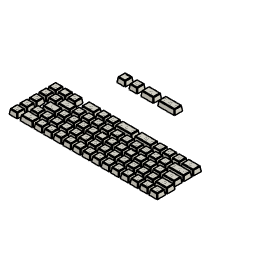
Launch Lite Keycaps v6 (Autodesk Fusion 360 design; units mm, degrees)
Autodesk Fusion 360 part; units mm, degrees
note: some values were not read from the file. Set by a fixed rule: which face or edge a step refers to.
sketch "Sketch1" plane through (0, 0, 0) normal (0, 0, 1) x (1, 0, 0)
  line L0 (-100, 50) -> (-82, 50)
  line L1 (-82, 50) -> (-82, 32)
  line L2 (-82, 32) -> (-100, 32)
  line L3 (-100, 32) -> (-100, 50)
  line L4 (-75, 50) -> (-57, 50)
  line L5 (-57, 50) -> (-57, 32)
  line L6 (-57, 32) -> (-75, 32)
  line L7 (-75, 32) -> (-75, 50)
  line L8 (-50, 50) -> (-23, 50)
  line L9 (-23, 50) -> (-23, 32)
  line L10 (-23, 32) -> (-50, 32)
  line L11 (-50, 32) -> (-50, 50)
  line L12 (-15, 50) -> (21, 50)
  line L13 (21, 50) -> (21, 32)
  line L14 (21, 32) -> (-15, 32)
  line L15 (-15, 32) -> (-15, 50)
  dimension "d1" = 18
  dimension "d2" = 18
  dimension "d3" = 18
  dimension "d4" = 18
  dimension "d5" = 27
  dimension "d6" = 18
  dimension "d7" = 36
  dimension "d8" = 18
  constraint horizontal L0
  constraint vertical L1
  constraint horizontal L2
  constraint vertical L3
  constraint horizontal L4
  constraint vertical L5
  constraint horizontal L6
  constraint vertical L7
  constraint horizontal L8
  constraint vertical L9
  constraint horizontal L10
  constraint vertical L11
  constraint horizontal L12
  constraint vertical L13
  constraint horizontal L14
  constraint vertical L15
  measures "d1" distance of L0.start L0.end
  measures "d2" distance of L0.start L2.end
  measures "d3" distance of L4.start L4.end
  measures "d4" distance of L4.start L6.end
  measures "d5" distance of L8.start L8.end
  measures "d6" distance of L8.start L10.end
  measures "d7" distance of L12.start L12.end
  measures "d8" distance of L12.start L14.end
extrude "Extrude1" add sketch "Sketch1" along normal blind 10 makes body 1 at (-41, 38, 0) makes body 2 at (-69, 44, 0) makes body 3 at (-3, 44, 0) makes body 4 at (-94, 44, 0)
shell "Shell1" thickness 1.75 removed faces 4 at (-41, 38, 10) at (-69, 44, 10) at (-3, 44, 10) at (-94, 44, 10) on bodies 1 2 3 4
sketch "Sketch2" plane through (0, 0, 1.75) normal (0, 0, 1) x (-1, 0, 0)
  line L0 (98.25, -33.75) -> (83.75, -33.75)
  line L1 (83.75, -33.75) -> (83.75, -48.25)
  line L2 (83.75, -48.25) -> (98.25, -48.25)
  line L3 (98.25, -48.25) -> (98.25, -33.75)
  circle A0 centre (91, -41) radius 2.8
  circle A1 centre (66, -41) radius 2.8
  circle A2 centre (36.5, -41) radius 2.8
  circle A3 centre (9, -41) radius 2.8
  circle A4 centre (-3, -41) radius 2.8
  circle A5 centre (-15, -41) radius 2.8
  dimension "d12" = 5.6
  dimension "d13" = 5.6
  dimension "d14" = 5.6
  dimension "d15" = 5.6
  dimension "d16" = 5.6
  dimension "d17" = 5.6
  measures "d12" diameter of A0
  measures "d13" diameter of A1
  measures "d14" diameter of A2
  measures "d15" diameter of A3
  measures "d16" diameter of A4
  measures "d17" diameter of A5
extrude "Extrude2" add sketch "Sketch2" along normal blind 8.2 contours A0 | A1 | A2 | A3 | A4 | A5 bodies 1 2 3 4
draft "Draft1" angle -8 neutral plane through (0, 0, 10) pull (0, 0, 1) 16 faces at (21, 44, 3.3333) (-3, 50, 3.3333) (-41, 50, 3.3333) (-69, 50, 3.3333) (-94, 50, 3.3333) (-82, 44, 3.3333) (-57, 44, 3.3333) (-23, 44, 3.3333) (9, 32, 3.3333) (-32, 32, 3.3333) (-63, 32, 3.3333) (-88, 32, 3.3333) (-15, 38, 3.3333) (-50, 38, 3.3333) (-75, 38, 3.3333) (-100, 38, 3.3333) on bodies 1 2 3 4
draft "Draft2" angle 8 neutral plane through (0, 0, 10) pull (0, 0, 1) 16 faces at (-24.75, 43.4167, 7.25) (-40.4167, 48.25, 4.5) (-32.5833, 33.75, 4.5) (8.4167, 33.75, 7.25) (19.25, 43.4167, 7.25) (-58.75, 43.4167, 7.25) (-63.5833, 33.75, 7.25) (-88.5833, 33.75, 7.25) (-83.75, 43.4167, 7.25) (-93.4167, 48.25, 7.25) (-98.25, 38.5833, 7.25) (-68.4167, 48.25, 7.25) (-73.25, 38.5833, 7.25) (-2.4167, 48.25, 7.25) (-13.25, 38.5833, 7.25) (-48.25, 38.5833, 7.25) on bodies 1 2 3 4
extrude "Extrude3" add sketch "Sketch2" along normal blind 2 contours L0 L1 L2 L3 bodies 1 2 3 4
sketch "Sketch3" plane through (0, 0, 9.95) normal (0, 0, 1) x (-1, 0, 0)
  circle A0 centre (-15, -41) radius 2.8
  line L0 (-15.625, -38.9) -> (-14.375, -38.9)
  line L1 (-14.375, -38.9) -> (-14.375, -43.15)
  line L2 (-14.375, -43.15) -> (-15.625, -43.15)
  line L3 (-15.625, -43.15) -> (-15.625, -38.9)
  line L4 (-12.925, -41.5) -> (-17.175, -41.5)
  line L5 (-12.925, -40.25) -> (-12.925, -41.5)
  line L6 (-17.175, -40.25) -> (-12.925, -40.25)
  line L7 (-17.175, -41.5) -> (-17.175, -40.25)
  line L8 (-0.875, -41.5) -> (-5.125, -41.5)
  line L9 (-5.125, -40.25) -> (-0.875, -40.25)
  line L10 (-2.375, -38.9) -> (-2.375, -43.15)
  line L11 (-3.625, -43.15) -> (-3.625, -38.9)
  line L12 (-5.125, -41.5) -> (-5.125, -40.25)
  line L13 (-3.625, -38.9) -> (-2.375, -38.9)
  line L14 (-0.875, -40.25) -> (-0.875, -41.5)
  line L15 (-2.375, -43.15) -> (-3.625, -43.15)
  line L16 (11.125, -41.5) -> (6.875, -41.5)
  line L17 (6.875, -40.25) -> (11.125, -40.25)
  line L18 (9.625, -38.9) -> (9.625, -43.15)
  line L19 (8.375, -43.15) -> (8.375, -38.9)
  line L20 (6.875, -41.5) -> (6.875, -40.25)
  line L21 (8.375, -38.9) -> (9.625, -38.9)
  line L22 (11.125, -40.25) -> (11.125, -41.5)
  line L23 (9.625, -43.15) -> (8.375, -43.15)
  line L24 (38.575, -41.5) -> (34.375, -41.5)
  line L25 (34.375, -40.3) -> (38.575, -40.3)
  line L26 (37.125, -38.9) -> (37.125, -43.15)
  line L27 (35.875, -43.15) -> (35.875, -38.9)
  line L28 (34.375, -41.5) -> (34.375, -40.3)
  line L29 (35.875, -38.9) -> (37.125, -38.9)
  line L30 (38.575, -40.3) -> (38.575, -41.5)
  line L31 (37.125, -43.15) -> (35.875, -43.15)
  line L32 (68.125, -41.5) -> (63.875, -41.5)
  line L33 (63.875, -40.25) -> (68.125, -40.25)
  line L34 (66.625, -38.9) -> (66.625, -43.15)
  line L35 (65.375, -43.15) -> (65.375, -38.9)
  line L36 (63.875, -41.5) -> (63.875, -40.25)
  line L37 (65.375, -38.9) -> (66.625, -38.9)
  line L38 (68.125, -40.25) -> (68.125, -41.5)
  line L39 (66.625, -43.15) -> (65.375, -43.15)
  line L40 (93.125, -41.5) -> (88.875, -41.5)
  line L41 (88.875, -40.25) -> (93.125, -40.25)
  line L42 (91.625, -38.9) -> (91.625, -43.15)
  line L43 (90.375, -43.15) -> (90.375, -38.9)
  line L44 (88.875, -41.5) -> (88.875, -40.25)
  line L45 (90.375, -38.9) -> (91.625, -38.9)
  line L46 (93.125, -40.25) -> (93.125, -41.5)
  line L47 (91.625, -43.15) -> (90.375, -43.15)
  dimension "d24" = 4.25
  dimension "d25" = 1.25
  dimension "d26" = 4.25
  dimension "d27" = 1.25
  dimension "d28" = 4.25
  dimension "d29" = 1.25
  dimension "d30" = 4.25
  dimension "d31" = 1.25
  dimension "d32" = 4.25
  dimension "d33" = 1.25
  dimension "d34" = 4.25
  dimension "d35" = 1.25
  dimension "d36" = 4.25
  dimension "d37" = 1.25
  dimension "d38" = 4.2
  dimension "d39" = 1.2
  dimension "d40" = 4.25
  dimension "d41" = 1.25
  dimension "d42" = 4.25
  dimension "d43" = 1.25
  dimension "d44" = 4.25
  dimension "d45" = 1.25
  dimension "d46" = 4.25
  dimension "d47" = 1.25
  constraint horizontal L0
  constraint vertical L1
  constraint horizontal L2
  constraint vertical L3
  constraint horizontal L13
  constraint vertical L10
  constraint horizontal L15
  constraint vertical L11
  constraint horizontal L21
  constraint vertical L18
  constraint horizontal L23
  constraint vertical L19
  constraint horizontal L29
  constraint vertical L26
  constraint horizontal L31
  constraint vertical L27
  constraint horizontal L37
  constraint vertical L34
  constraint horizontal L39
  constraint vertical L35
  constraint horizontal L45
  constraint vertical L42
  constraint horizontal L47
  constraint vertical L43
  measures "d24" distance of L0.start L2.end
  measures "d25" distance of L1 L3
  measures "d26" distance of L5.start L6.start
  measures "d27" distance of L4 L6
  measures "d28" distance of L11.end L11.start
  measures "d29" distance of L10 L11
  measures "d30" distance of L9.start L9.end
  measures "d31" distance of L8 L9
  measures "d32" distance of L19.end L19.start
  measures "d33" distance of L18 L19
  measures "d34" distance of L17.start L17.end
  measures "d35" distance of L16 L17
  measures "d36" distance of L27.end L27.start
  measures "d37" distance of L26 L27
  measures "d38" distance of L25.start L25.end
  measures "d39" distance of L24 L25
  measures "d40" distance of L35.end L35.start
  measures "d41" distance of L34 L35
  measures "d42" distance of L33.start L33.end
  measures "d43" distance of L32 L33
  measures "d44" distance of L43.end L43.start
  measures "d45" distance of L42 L43
  measures "d46" distance of L41.start L41.end
  measures "d47" distance of L40 L41
extrude "Extrude4" cut sketch "Sketch3" against normal blind 8 contours L0 L1 L3 L6 | L1 L3 L4 L6 | L3 L4 L6 L7 | L1 L4 L5 L6 | L1 L2 L3 L4 | L8 L9 L10 L14 | L8 L10 L11 L15 | L8 L9 L10 L11 | L8 L9 L11 L12 | L9 L10 L11 L13 | L16 L17 L18 L22 | L16 L18 L19 L23 | L16 L17 L18 L19 | L16 L17 L19 L20 | L17 L18 L19 L21 | L24 L25 L26 L30 | L24 L26 L27 L31 | L24 L25 L26 L27 | L24 L25 L27 L28 | L25 L26 L27 L29 | L32 L33 L34 L38 | L32 L34 L35 L39 | L32 L33 L34 L35 | L32 L33 L35 L36 | L33 L34 L35 L37 | L40 L41 L42 L46 | L40 L42 L43 L47 | L40 L41 L42 L43 | L40 L41 L43 L44 | L41 L42 L43 L45 bodies 1 2 3 4
move_body "Move1" bodies 1 3 2 4 to x (1, 0, 0) y (0, -1, 0) z (0, 0, -1) at (0, 83, 10)
fillet "Fillet2" radius 1.25 31 edges at (-49.2973, 50.2973, 5) (-23.7027, 50.2973, 5) (-23.7027, 33.7027, 5) (-36.5, 49.5946, 10) (-24.4054, 42, 10) (-49.2973, 33.7027, 5) (-36.5, 34.4054, 10) (-48.5946, 42, 10) (-74.2973, 50.2973, 5) (-57.7027, 50.2973, 5) (-57.7027, 33.7027, 5) (-58.4054, 42, 10) (-66, 49.5946, 10) (-74.2973, 33.7027, 5) (-73.5946, 42, 10) (-66, 34.4054, 10) (-14.2973, 50.2973, 5) (20.2973, 50.2973, 5) (3, 49.5946, 10) (19.5946, 42, 10) (20.2973, 33.7027, 5) (-14.2973, 33.7027, 5) (-13.5946, 42, 10) (3, 34.4054, 10) (-99.2973, 50.2973, 5) (-91, 49.5946, 10) (-83.4054, 42, 10) (-82.7027, 50.2973, 5) (-91, 34.4054, 10) (-98.5946, 42, 10) (-99.2973, 33.7027, 5) on bodies 1 2 3 4
fillet "Fillet2" radius 1.25 1 edges at (-82.7027, 33.7027, 5) on bodies 1 2 3 4
sketch "Sketch4" plane through (0, 0, 10) normal (0, 0, 1) x (-1, 0, 0)
  line L0 (95, -47) -> (87, -47)
  line L1 (87, -47) -> (87, -48)
  line L2 (87, -48) -> (95, -48)
  line L3 (95, -48) -> (95, -47)
  line L4 (-18.508, -48.508) -> (12.508, -48.508)
  line L5 (12.508, -48.508) -> (12.508, -35.492)
  line L6 (12.508, -35.492) -> (-18.508, -35.492)
  line L7 (-18.508, -35.492) -> (-18.508, -48.508)
  line L8 (25.492, -48.508) -> (47.508, -48.508)
  line L9 (47.508, -48.508) -> (47.508, -35.492)
  line L10 (47.508, -35.492) -> (25.492, -35.492)
  line L11 (25.492, -35.492) -> (25.492, -48.508)
  line L12 (84.492, -48.508) -> (97.508, -48.508)
  line L13 (97.508, -48.508) -> (97.508, -35.492)
  line L14 (97.508, -35.492) -> (84.492, -35.492)
  line L15 (84.492, -35.492) -> (84.492, -48.508)
  line L16 (59.492, -48.508) -> (72.508, -48.508)
  line L17 (72.508, -48.508) -> (72.508, -35.492)
  line L18 (72.508, -35.492) -> (59.492, -35.492)
  line L19 (59.492, -35.492) -> (59.492, -48.508)
  dimension "d50" = 8
  constraint horizontal L0
  constraint vertical L1
  constraint horizontal L2
  constraint vertical L3
  measures "d50" distance of L0.start L0.end
extrude "Extrude5" add sketch "Sketch4" along normal blind 0.3 contours L0 L1 L2 L3 bodies 4
fillet "Fillet1" radius 0.29 8 edges at (-91, 48, 10.3) (-87, 48, 10.15) (-87, 47, 10.15) (-87, 47.5, 10.3) (-91, 47, 10.3) (-95, 48, 10.15) (-95, 47.5, 10.3) (-95, 47, 10.15) on bodies 4
copy_body "CopyPasteBodies1" bodies 3 makes body 5
move_body "Move2" bodies 5 to x (1, 0, 0) y (0, 1, 0) z (0, 0, 1) at (40, -90, 0)
copy_body "CopyPasteBodies2" bodies 3 makes body 6
move_body "Move3" bodies 6 to x (1, 0, 0) y (0, 1, 0) z (0, 0, 1) at (0, -90, 0)
copy_body "CopyPasteBodies3" bodies 2 makes body 7
move_body "Move4" bodies 7 to x (1, 0, 0) y (0, 1, 0) z (0, 0, 1) at (40, -90, 0)
copy_body "CopyPasteBodies4" bodies 2 makes body 8
move_body "Move5" bodies 8 to x (1, 0, 0) y (0, 1, 0) z (0, 0, 1) at (20, -90, 0)
copy_body "CopyPasteBodies5" bodies 1 makes body 9
move_body "Move6" bodies 9 to x (1, 0, 0) y (0, 1, 0) z (0, 0, 1) at (-35, -90, 0)
copy_body "CopyPasteBodies6" bodies 2 makes body 10
move_body "Move7" bodies 10 to x (1, 0, 0) y (0, 1, 0) z (0, 0, 1) at (-40, -90, 0)
copy_body "CopyPasteBodies8" bodies 4 makes body 11
move_body "Move8" bodies 11 to x (1, 0, 0) y (0, 1, 0) z (0, 0, 1) at (-35, -90, 0)
copy_body "CopyPasteBodies9" bodies 2 makes body 12
move_body "Move9" bodies 12 to x (1, 0, 0) y (0, 1, 0) z (0, 0, 1) at (-80, -90, 0)
copy_body "CopyPasteBodies10" bodies 2 makes body 13
move_body "Move10" bodies 13 to x (1, 0, 0) y (0, 1, 0) z (0, 0, 1) at (-60, -110, 0)
copy_body "CopyPasteBodies11" bodies 2 makes body 14
move_body "Move11" bodies 14 to x (1, 0, 0) y (0, 1, 0) z (0, 0, 1) at (138, -90, 0)
copy_body "CopyPasteBodies12" bodies 2 makes body 15
move_body "Move12" bodies 15 to x (1, 0, 0) y (0, 1, 0) z (0, 0, 1) at (158, -90, 0)
copy_body "CopyPasteBodies13" bodies 2 makes body 16
move_body "Move13" bodies 16 to x (1, 0, 0) y (0, 1, 0) z (0, 0, 1) at (178, -90, 0)
copy_body "CopyPasteBodies14" bodies 1 makes body 17
move_body "Move14" bodies 17 to x (1, 0, 0) y (0, 1, 0) z (0, 0, 1) at (173, -90, 0)
copy_body "CopyPasteBodies15" bodies 3 makes body 18
move_body "Move15" bodies 18 to x (1, 0, 0) y (0, 1, 0) z (0, 0, 1) at (129, -110, 0)
copy_body "CopyPasteBodies16" bodies 14 15 16 makes body 19 makes body 20 makes body 21
move_body "Move16" bodies 19 20 21 to x (1, 0, 0) y (0, 1, 0) z (0, 0, 1) at (-9, -20, 0)
copy_body "CopyPasteBodies17" bodies 14 15 16 makes body 22 makes body 23 makes body 24
move_body "Move17" bodies 22 23 24 to x (1, 0, 0) y (0, 1, 0) z (0, 0, 1) at (-69, -20, 0)
copy_body "CopyPasteBodies18" bodies 14 15 16 makes body 25 makes body 26 makes body 27
move_body "Move18" bodies 25 26 27 to x (1, 0, 0) y (0, 1, 0) z (0, 0, 1) at (-129, -20, 0)
copy_body "CopyPasteBodies19" bodies 2 makes body 28
move_body "Move19" bodies 28 to x (1, 0, 0) y (0, 1, 0) z (0, 0, 1) at (-11, -110, 0)
copy_body "CopyPasteBodies20" bodies 1 makes body 29
move_body "Move20" bodies 29 to x (1, 0, 0) y (0, 1, 0) z (0, 0, 1) at (-65, -110, 0)
copy_body "CopyPasteBodies21" bodies 1 makes body 30
move_body "Move21" bodies 30 to x (1, 0, 0) y (0, 1, 0) z (0, 0, 1) at (173, -130, 0)
copy_body "CopyPasteBodies24" bodies 2 makes body 31
move_body "Move25" bodies 31 to x (1, 0, 0) y (0, 1, 0) z (0, 0, 1) at (-80, -110, 0)
copy_body "CopyPasteBodies25" bodies 2 makes body 32
move_body "Move26" bodies 32 to x (1, 0, 0) y (0, 1, 0) z (0, 0, 1) at (-80, -130, 0)
copy_body "CopyPasteBodies26" bodies 2 makes body 33
move_body "Move27" bodies 33 to x (1, 0, 0) y (0, 1, 0) z (0, 0, 1) at (178, -130, 0)
copy_body "CopyPasteBodies27" bodies 2 makes body 34
move_body "Move28" bodies 34 to x (1, 0, 0) y (0, 1, 0) z (0, 0, 1) at (158, -130, 0)
copy_body "CopyPasteBodies28" bodies 2 makes body 35
move_body "Move29" bodies 35 to x (1, 0, 0) y (0, 1, 0) z (0, 0, 1) at (138, -130, 0)
copy_body "CopyPasteBodies29" bodies 4 makes body 36
move_body "Move30" bodies 36 to x (1, 0, 0) y (0, 1, 0) z (0, 0, 1) at (143, -130, 0)
copy_body "CopyPasteBodies30" bodies 2 makes body 37
move_body "Move31" bodies 37 to x (1, 0, 0) y (0, 1, 0) z (0, 0, 1) at (98, -130, 0)
copy_body "CopyPasteBodies31" bodies 2 makes body 38
move_body "Move32" bodies 38 to x (1, 0, 0) y (0, 1, 0) z (0, 0, 1) at (78, -130, 0)
copy_body "CopyPasteBodies32" bodies 4 makes body 39
move_body "Move33" bodies 39 to x (1, 0, 0) y (0, 1, 0) z (0, 0, 1) at (83, -130, 0)
copy_body "CopyPasteBodies33" bodies 2 makes body 40
move_body "Move34" bodies 40 to x (1, 0, 0) y (0, 1, 0) z (0, 0, 1) at (38, -130, 0)
copy_body "CopyPasteBodies34" bodies 2 makes body 41
move_body "Move35" bodies 41 to x (1, 0, 0) y (0, 1, 0) z (0, 0, 1) at (18, -130, 0)
copy_body "CopyPasteBodies35" bodies 2 makes body 42
move_body "Move36" bodies 42 to x (1, 0, 0) y (0, 1, 0) z (0, 0, 1) at (-2, -130, 0)
copy_body "CopyPasteBodies36" bodies 2 makes body 43
move_body "Move37" bodies 43 to x (1, 0, 0) y (0, 1, 0) z (0, 0, 1) at (-22, -130, 0)
copy_body "CopyPasteBodies37" bodies 1 makes body 44
move_body "Move38" bodies 44 to x (1, 0, 0) y (0, 1, 0) z (0, 0, 1) at (-76, -130, 0)
copy_body "CopyPasteBodies38" bodies 1 makes body 45
move_body "Move39" bodies 45 to x (1, 0, 0) y (0, 1, 0) z (0, 0, 1) at (178, -150, 0)
copy_body "CopyPasteBodies39" bodies 2 makes body 46
move_body "Move40" bodies 46 to x (1, 0, 0) y (0, 1, 0) z (0, 0, 1) at (183, -150, 0)
copy_body "CopyPasteBodies40" bodies 46 makes body 47
move_body "Move41" bodies 47 to x (1, 0, 0) y (0, 1, 0) z (0, 0, 1) at (-20, 0, 0)
copy_body "CopyPasteBodies41" bodies 46 makes body 48
move_body "Move42" bodies 48 to x (1, 0, 0) y (0, 1, 0) z (0, 0, 1) at (-40, 0, 0)
copy_body "CopyPasteBodies42" bodies 46 makes body 49
move_body "Move43" bodies 49 to x (1, 0, 0) y (0, 1, 0) z (0, 0, 1) at (-60, 0, 0)
copy_body "CopyPasteBodies43" bodies 46 makes body 50
move_body "Move44" bodies 50 to x (1, 0, 0) y (0, 1, 0) z (0, 0, 1) at (-80, 0, 0)
copy_body "CopyPasteBodies44" bodies 46 makes body 51
move_body "Move45" bodies 51 to x (1, 0, 0) y (0, 1, 0) z (0, 0, 1) at (-100, 0, 0)
copy_body "CopyPasteBodies45" bodies 46 makes body 52
move_body "Move46" bodies 52 to x (1, 0, 0) y (0, 1, 0) z (0, 0, 1) at (-120, 0, 0)
copy_body "CopyPasteBodies46" bodies 46 makes body 53
move_body "Move47" bodies 53 to x (1, 0, 0) y (0, 1, 0) z (0, 0, 1) at (-140, 0, 0)
copy_body "CopyPasteBodies47" bodies 46 makes body 54
move_body "Move48" bodies 54 to x (1, 0, 0) y (0, 1, 0) z (0, 0, 1) at (-160, 0, 0)
copy_body "CopyPasteBodies48" bodies 46 makes body 55
move_body "Move49" bodies 55 to x (1, 0, 0) y (0, 1, 0) z (0, 0, 1) at (-180, 0, 0)
copy_body "CopyPasteBodies49" bodies 46 makes body 56
move_body "Move50" bodies 56 to x (1, 0, 0) y (0, 1, 0) z (0, 0, 1) at (-200, 0, 0)
copy_body "CopyPasteBodies50" bodies 46 makes body 57
move_body "Move51" bodies 57 to x (1, 0, 0) y (0, 1, 0) z (0, 0, 1) at (-220, 0, 0)
copy_body "CopyPasteBodies51" bodies 46 makes body 58
move_body "Move52" bodies 58 to x (1, 0, 0) y (0, 1, 0) z (0, 0, 1) at (-240, 0, 0)
copy_body "CopyPasteBodies52" bodies 46 makes body 59
move_body "Move53" bodies 59 to x (1, 0, 0) y (0, 1, 0) z (0, 0, 1) at (-263, 0, 0)
copy_body "CopyPasteBodies53" bodies 2 makes body 60
move_body "Move54" bodies 60 to x (1, 0, 0) y (0, 1, 0) z (0, 0, 1) at (212, -170, 0)
copy_body "CopyPasteBodies54" bodies 60 makes body 61
move_body "Move55" bodies 61 to x (1, 0, 0) y (0, 1, 0) z (0, 0, 1) at (-20, 0, 0)
copy_body "CopyPasteBodies55" bodies 60 makes body 62
move_body "Move56" bodies 62 to x (1, 0, 0) y (0, 1, 0) z (0, 0, 1) at (-40, 0, 0)
copy_body "CopyPasteBodies56" bodies 60 makes body 63
move_body "Move57" bodies 63 to x (1, 0, 0) y (0, 1, 0) z (0, 0, 1) at (-60, 0, 0)
copy_body "CopyPasteBodies57" bodies 60 makes body 64
move_body "Move58" bodies 64 to x (1, 0, 0) y (0, 1, 0) z (0, 0, 1) at (-80, 0, 0)
copy_body "CopyPasteBodies58" bodies 60 62 61 63 64 makes body 65 makes body 66 makes body 67 makes body 68 makes body 69
move_body "Move59" bodies 65 66 67 68 69 to x (1, 0, 0) y (0, 1, 0) z (0, 0, 1) at (-100, 0, 0)
copy_body "CopyPasteBodies59" bodies 69 makes body 70
move_body "Move60" bodies 70 to x (1, 0, 0) y (0, 1, 0) z (0, 0, 1) at (-20, 0, 0)
copy_body "CopyPasteBodies60" bodies 69 makes body 71
move_body "Move61" bodies 71 to x (1, 0, 0) y (0, 1, 0) z (0, 0, 1) at (-40, 0, 0)
copy_body "CopyPasteBodies61" bodies 69 makes body 72
move_body "Move62" bodies 72 to x (1, 0, 0) y (0, 1, 0) z (0, 0, 1) at (-60, 0, 0)
copy_body "CopyPasteBodies62" bodies 1 makes body 73
move_body "Move63" bodies 73 to x (1, 0, 0) y (0, 1, 0) z (0, 0, 1) at (-82, -170, 0)
copy_body "CopyPasteBodies63" bodies 2 makes body 74
move_body "Move64" bodies 74 to x (1, 0, 0) y (0, 1, 0) z (0, 0, 1) at (-80, -170, 0)
named bodies: "2U", "1U", "3U", "1U w/ bar", "Spacebar", "Left Space", "Spacebar (1)", "Right Space", "Right  Alt", "1U (1)", "Right Ctrl", "Right Fn", "1U (2)", "Left", "Down", "1U (4)", "Right", "1U (5)", "UP", "1U (6)", "Super", "1U (7)", "Left Fn", "1U (8)", "Alt", "2U (1)", "Ctrl", "Left shift", "1U (6) (1)", "1U (7) (1)", "1U (8) (1)", "1U (6) (2)", "1U (7) (2)", "1U (8) (2)", "1U (6) (3)", "1U (7) (3)", "1U (8) (3)", ".>", ",<", "1U (9)", "/?", "2U (2)", "Right shift", "2U (3)", "Caps", "1U (11)", "End", "1U (12)", "End (1)", "1U (10)", "1U (13)", "1U (14)", "1U w/ bar (1)", "1U (15)", "1U (16)", "1U w/ bar (2)", "1U (17)", "1U (18)", "1U (19)", ":;", "1U (20)", "'\"", "2U (4)", "Enter", "2U (5)", "Tab", "1U (21)", "1U (21) (1)", "1U (21) (2)", "1U (21) (3)", "1U (21) (4)", "1U (21) (5)", "1U (21) (6)", "1U (21) (7)", "1U (21) (8)", "1U (21) (9)", "1U (21) (10)", "[{", "1U (21) (11)", "]}", "1U (21) (12)", "\\|", "1U (21) (13)", "PgUp", "1U (22)", "Esc", "1U (22) (1)", "1U (22) (2)", "1U (22) (3)", "1U (22) (4)", "1U (22) (5)", "1U (22) (2) (1)", "1U (22) (1) (1)", "1U (22) (3) (1)", "1U (22) (4) (1)", "1U (22) (4) (1) (1)", "1U (22) (4) (1) (2)", "1U (22) (4) (1) (3)", "2U (6)", "Delete", "1U (23)", "Home"
